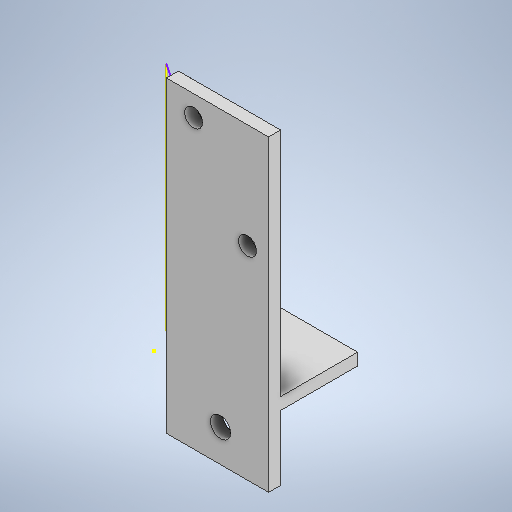
# Autodesk Inventor part: SolenoidMount
Saved by Autodesk Inventor 2025.1 (Build 291241000, 241)
## iProperties
Created: 2025-11-05
Part Number: SolenoidMount
Material: Generic
Document SubType Name: Modeling
Designer: Juxin
Density: 1 g/cm^3
Appearance: Default
Author: Juxin
Autodesk Inventor part; units mm, degrees
ref_plane "YZ Plane" through (0, 0, 0) normal (1, 0, 0) x (0, 1, 0)
ref_plane "XZ Plane" through (0, 0, 0) normal (0, 1, 0) x (-1, 0, 0)
ref_plane "XY Plane" through (0, 0, 0) normal (0, 0, 1) x (1, 0, 0)
sketch "Sketch1" plane through (0, 0, 0) normal (0, 1, 0) x (-1, 0, 0)
  line L0 (0, 0) -> (25.4, 0)
  line L1 (25.4, 0) -> (25.4, -20.32)
  line L2 (25.4, -20.32) -> (0, -20.32)
  line L3 (0, -20.32) -> (0, 0)
  dimension "d0" = 25.4
  dimension "d1" = 20.32
  constraints: 8 end point, 2 parallel, 1 horizontal, 1 perpendicular
  measures "d0" distance of L1.end L2.end
  measures "d1" distance of L0.end L1.end
extrude "Extrusion1" add sketch "Sketch1" along normal blind 3.1623
sketch "Sketch2" plane through (0, 0, 0) normal (0, -1, 0) x (1, 0, 0)
  line L0 (-25.4, 0) -> (0, 0) projected
  line L1 (0, 0) -> (0, -20.32) projected
  line L2 (-25.4, 0) -> (0, 0)
  line L3 (0, 0) -> (0, -3.175)
  line L4 (0, -3.175) -> (-25.4, -3.175)
  line L5 (-25.4, -3.175) -> (-25.4, 0)
  dimension "d4" = 3.175
  constraints: 8 end point, 2 parallel, 1 horizontal, 1 perpendicular, 1 point on line
  measures "d4" distance of L2.end L3.end
extrude "Extrusion2" add sketch "Sketch2" along normal blind 17.145
sketch "Sketch3" plane through (0, 3.1623, 0) normal (0, 1, 0) x (1, 0, 0)
  line L0 (-25.4, 0) -> (0, 0) projected
  line L1 (0, 0) -> (0, 20.32) projected
  line L2 (-25.4, 0) -> (0, 0)
  line L3 (0, 0) -> (0, 3.175)
  line L4 (0, 3.175) -> (-25.4, 3.175)
  line L5 (-25.4, 3.175) -> (-25.4, 0)
  dimension "d7" = 3.175
  constraints: 8 end point, 2 parallel, 1 horizontal, 1 perpendicular, 1 point on line
  measures "d7" distance of L3.end L2.end
extrude "Extrusion3" add sketch "Sketch3" along normal blind 60.96
sketch "Sketch4" plane through (0, 3.1623, -3.175) normal (0, 0, -1) x (-1, 0, 0)
  line L0 (0, 60.96) -> (25.4, 60.96) projected
  line L1 (25.4, 60.96) -> (19.812, 60.96)
  line L2 (0, 60.96) -> (9.271, 60.96)
  line L3 (0, 0) -> (25.4, 0) projected
  line L4 (12.7, 0) -> (12.7, 60.96)
  line L5 (12.7, 0) -> (22.733, 0) construction
  line L6 (12.7, 0) -> (2.667, 0) construction
  line L7 (2.667, 0) -> (2.667, 60.96) construction
  line L8 (22.733, 0) -> (22.733, 60.96) construction
  line L9 (25.4, 60.96) -> (0, 60.96) construction
  line L10 (2.667, 60.96) -> (2.667, 21.59) construction
  line L11 (2.667, 21.59) -> (22.733, 21.59) construction
  line L12 (2.667, 60.96) -> (5.588, 60.96) construction
  line L13 (5.588, 60.96) -> (5.588, 21.59) construction
  line L14 (22.733, 60.96) -> (19.812, 60.96) construction
  line L15 (19.812, 60.96) -> (19.812, 21.59) construction
  line L16 (22.733, 60.96) -> (22.733, 55.499) construction
  line L17 (22.733, 55.499) -> (19.812, 55.499) construction
  line L18 (2.667, 21.59) -> (2.667, 33.274) construction
  line L19 (2.667, 33.274) -> (5.588, 33.274) construction
  circle A0 centre (19.812, 55.499) radius 2.3813
  circle A1 centre (5.588, 33.274) radius 2.3813
  point P0 (0, -3.1623)
  dimension "d76" = 10.033
  dimension "d77" = 10.033
  dimension "d78" = 39.37
  dimension "d79" = 2.921
  dimension "d80" = 2.921
  dimension "d81" = 5.461
  dimension "d82" = 11.684
  dimension "d83" = 4.7625
  dimension "d84" = 4.7625
  constraints: 34 end point, 13 point on line, 6 perpendicular, 2 centre point, 2 coincident, 2 midpoint, 1 parallel, 4 other
  measures "d76" distance of L4.start L5.end
  measures "d77" distance of L4.start L6.end
  measures "d78" distance of L7.end L10.end
  measures "d79" distance of L7.end L12.end
  measures "d80" distance of L8.end L14.end
  measures "d81" distance of L8.end L16.end
  measures "d82" distance of L10.end L18.end
  measures "d83" diameter of A0
  measures "d84" diameter of A1
extrude "Extrusion4" cut sketch "Sketch4" against normal blind 63.5
sketch "Sketch7" plane through (0, 0, -3.175) normal (0, 0, -1) x (-1, 0, 0)
  line L0 (25.4, -17.145) -> (0, -17.145) projected
  line L1 (12.7, -17.145) -> (12.7, -8.5725)
  circle A0 centre (12.7, -8.5725) radius 2.667
  point P0 (0, 0)
  dimension "d23" = 5.334
  constraints: 2 end point, 1 centre point, 1 coincident, 1 midpoint, 1 vertical
  measures "d23" diameter of A0
extrude "Extrusion7" cut sketch "Sketch7" against normal blind 46.0375
move faces "Move1" translate (0, 0, -3.175) faces at (-8.4667, 1.0541, -20.32)
move faces "Move11" translate (-4.7625, 0, 0) faces at (-25.4, 16.7132, -1.0583)
move faces "Move13" translate (1.5875, 0, 0) faces at (-30.1625, 16.7132, -1.0583)
move faces "Move14" translate (1.6002, 0, 0) faces at (-28.575, 16.7132, -1.0583)
sketch "Sketch16" plane through (-30.1625, 0, -23.495) normal (-1, 0, 0) x (0, 0, 1)
  line L0 (0, 3.1623) -> (20.32, 3.1623) projected
  line L1 (20.32, 3.1623) -> (20.32, 64.1223) projected
  line L2 (0, 3.1623) -> (20.32, 3.1623)
  line L3 (20.32, 3.1623) -> (20.32, 64.1223)
  line L4 (20.32, 64.1223) -> (0, 3.1623)
  point P0 (23.495, 0)
  constraints: 6 end point, 2 perpendicular
extrude "Extrusion18" add sketch "Sketch16" against normal blind 6.35
extrude "Extrusion19" cut sketch "Sketch16" against normal blind 3.175
body "Solid1"
